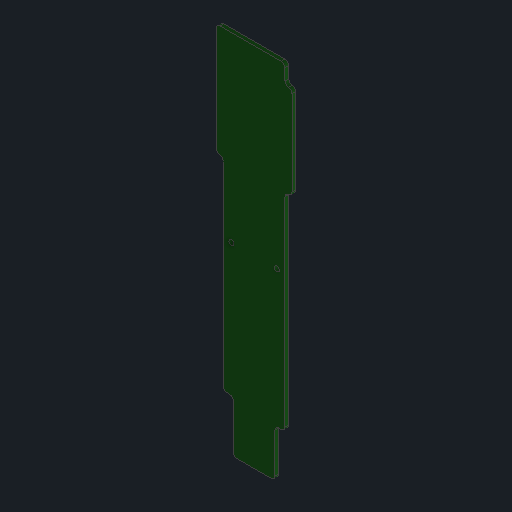
# Autodesk Inventor part: Power Board
Saved by Autodesk Inventor 2026.1 (Build 301233020, 233B)
## iProperties
Created: 2025-11-16
Part Number: Power Board
Material: Generic
Document SubType Name: Modeling
Designer: Bahaa
Density: 1 g/cm^3
Appearance: Default
Author: Bahaa
Autodesk Inventor part; units mm, degrees
ref_plane "YZ Plane" through (0, 0, 0) normal (1, 0, 0) x (0, 1, 0)
ref_plane "XZ Plane" through (0, 0, 0) normal (0, 1, 0) x (-1, 0, 0)
ref_plane "XY Plane" through (0, 0, 0) normal (0, 0, 1) x (1, 0, 0)
sketch "Sketch1" plane through (0, 0, 0) normal (0, 1, 0) x (-1, 0, 0)
  line L0 (-16.25, 55) -> (16.25, 55)
  line L1 (16.25, 55) -> (16.25, -55)
  line L2 (16.25, -55) -> (-16.25, -55)
  line L3 (-16.25, -55) -> (-16.25, 55)
  line L4 (-16.25, 55) -> (16.25, -55) construction
  line L5 (16.25, 55) -> (-16.25, -55) construction
  line L6 (16.25, 0) -> (12, 0) construction
  circle A0 centre (12, 0) radius 1.35
  line L7 (0, 0) -> (0, -55) construction
  circle A1 centre (-12, 0) radius 1.35
  line L8 (16.25, -55) -> (20, -55)
  line L9 (20, -55) -> (20, -37)
  line L10 (20, -37) -> (16.25, -37)
  line L11 (16.25, -37) -> (16.25, -55)
  line L12 (16.25, 0) -> (-16.25, 0) construction
  line L13 (0, 0) -> (0, 55) construction
  line L14 (-16.25, -55) -> (-20, -55)
  line L15 (-20, -55) -> (-20, -37)
  line L16 (-20, -37) -> (-16.25, -37)
  line L17 (-16.25, -37) -> (-16.25, -55)
  line L18 (16.25, 55) -> (-16.25, 55)
  line L19 (16.25, 55) -> (20, 55)
  line L20 (20, 55) -> (20, 37)
  line L21 (20, 37) -> (16.25, 37)
  line L22 (16.25, 37) -> (16.25, 55)
  line L23 (-20, 37) -> (-16.25, 37)
  line L24 (-16.25, 55) -> (-20, 55)
  line L25 (-20, 55) -> (-20, 37)
  line L26 (-16.25, 37) -> (-16.25, 55)
  circle A2 centre (12, 0) radius 2.55
  circle A3 centre (-12, 0) radius 2.55
  line L27 (20, 55) -> (-20, 55)
  line L28 (-20, 55) -> (-20, 90)
  line L29 (-20, 90) -> (20, 90)
  line L30 (20, 90) -> (20, 55)
  line L31 (16.25, 0) -> (-16.25, 0) construction
  line L32 (-20, -55) -> (-20, -90)
  line L33 (-20, -90) -> (20, -90)
  line L34 (20, -90) -> (20, -55)
  line L35 (16.25, -90) -> (16.25, 90)
  line L36 (-16.25, -90) -> (-16.25, 90)
  line L37 (20, -79.75) -> (-20, -79.75)
  line L38 (-11, -90) -> (11, -90)
  line L39 (11, -90) -> (11, -79.75)
  line L40 (11, -79.75) -> (-11, -79.75)
  line L41 (-11, -79.75) -> (-11, -90)
  line L42 (-11, -90) -> (11, -79.75) construction
  line L43 (11, -90) -> (-11, -79.75) construction
  line L44 (11, -87.25) -> (-11, -87.25)
  line L45 (0, 90) -> (0, 96) construction
  line L46 (20, 90) -> (-20, 90)
  line L47 (-20, 90) -> (-20, 96)
  line L48 (-20, 96) -> (20, 96)
  line L49 (20, 96) -> (20, 90)
  line L50 (-20, 90) -> (-16.25, 90)
  line L51 (-16.25, 90) -> (-16.25, 86)
  line L52 (-16.25, 86) -> (-20, 86)
  line L53 (-20, 86) -> (-20, 90)
  line L54 (-16.25, 90) -> (-16.25, 96)
  line L55 (-16.25, -79.75) -> (-11, -79.75)
  line L56 (-11, -79.75) -> (-11, -72.25)
  line L57 (-11, -72.25) -> (-16.25, -72.25)
  line L58 (-16.25, -72.25) -> (-16.25, -79.75)
  line L59 (20, 96) -> (16.25, 96)
  line L60 (16.25, 96) -> (16.25, 86)
  line L61 (16.25, 86) -> (20, 86)
  line L62 (20, 86) -> (20, 96)
  line L63 (16.25, -79.75) -> (11, -79.75)
  line L64 (11, -79.75) -> (11, -69.75)
  line L65 (11, -69.75) -> (16.25, -69.75)
  line L66 (16.25, -69.75) -> (16.25, -79.75)
  line L67 (20, -90) -> (-20, -90)
  line L68 (-20, -90) -> (-20, -97.25)
  line L69 (-20, -97.25) -> (20, -97.25)
  line L70 (20, -97.25) -> (20, -90)
  line L71 (11, -90) -> (11, -97.25)
  line L72 (-11, -90) -> (-11, -97.25)
  point P0 (16.25, 37)
  point P1 (-16.25, 37)
  point P2 (-16.25, -37)
  point P3 (16.25, -37)
  point P4 (-20, 55)
  point P5 (-20, -55)
  point P6 (0, 0)
  point P7 (0, -84.875)
  point P8 (-16.25, 86)
  point P9 (-20, 86)
  dimension "d10" = 32.5
  dimension "d11" = 110
  dimension "d16" = 2.7
  dimension "d30" = 18
  dimension "d34" = 5.1
  dimension "d35" = 40
  dimension "d36" = 35
  dimension "d39" = 40
  dimension "d40" = 24
  dimension "d41" = 10.25
  dimension "d43" = 5.125
  dimension "d45" = 2.75
  dimension "d46" = 11
  dimension "d47" = 20
  dimension "d48" = 6
  dimension "d49" = 40
  dimension "d50" = 6
  dimension "d51" = 3.75
  dimension "d52" = 4
  dimension "d53" = 5.25
  dimension "d54" = 7.5
  dimension "d55" = 3.75
  dimension "d56" = 10
  dimension "d57" = 5.25
  dimension "d58" = 10
  dimension "d59" = 7.25
  constraints: 146 end point, 20 parallel, 17 point on line, 16 symmetric about line, 15 perpendicular, 11 horizontal, 10 midpoint, 4 centre point, 2 coincident, 1 vertical, 2 other
  measures "d10" distance of L1.end L2.end
  measures "d11" distance of L0.end L1.end
  measures "d16" diameter of A0
  measures "d30" distance of L8.end L9.end
  measures "d34" diameter of A2
  measures "d35" distance of L28.end L29.end
  measures "d36" distance of L27.end L28.end
  measures "d39" diameter of L9 L7
  measures "d40" diameter of L6.end point (0, 0)
  measures "d41" distance between parallel lines of L33 L37
  measures "d43" distance from line of L33 point (0, -84.875)
  measures "d45" distance between parallel lines of L33 L44
  measures "d46" distance from line of point (0, -84.875) L39
  measures "d47" distance from line of L34 point (0, -84.875)
  measures "d48" distance of L45.start L45.end
  measures "d49" distance of L47.end L48.end
  measures "d50" distance of L48.end L29.end
  measures "d51" distance of L51.end L52.end
  measures "d52" distance of L50.end L51.end
  measures "d53" distance of L57.end L56.end
  measures "d54" distance of L56.end L55.end
  measures "d55" distance of L61.end L60.end
  measures "d56" distance of L60.end L59.end
  measures "d57" distance of L64.end L65.end
  measures "d58" distance of L63.end L64.end
  measures "d59" distance of L69.end L34.start
extrude "Extrusion1" add sketch "Sketch1" along normal blind 2 contours L36 L29 L35 L0 | L0 L1 L2 L3 | L3 L23 L25 L24 | L24 L28 L52 L36 | L19 L20 L21 L1 | L35 L61 L30 L19 | L35 L29 L30 L61 | L54 L48 L60 L29 | L60 L48 L49 L29 | L2 L35 L65 L64 L37 L56 L57 L36 | L37 L39 L44 L41 | L41 L44 L39 L33 | L33 L71 L69 L72 | A2 | A3
sketch "Sketch2" plane through (0, 0, 0) normal (0, -1, 0) x (1, 0, 0)
  line L0 (-16.25, -33.5) -> (-16.25, 37) projected
  line L1 (-16.25, -20.3135) -> (-16.25, -7.8135)
  line L2 (-16.25, -20.3135) -> (-7.5, -20.3135)
  line L3 (-7.5, -20.3135) -> (-7.5, -7.8135)
  line L4 (-7.5, -7.8135) -> (-16.25, -7.8135)
  line L5 (-16.25, -7.8135) -> (-16.25, -20.3135)
  line L6 (0, 0) -> (-16.25, 1.75) construction
  line L7 (0, 0) -> (0, 10) construction
  line L8 (0, 0) -> (-9.9425, 1.0707) construction
  line L9 (16.25, -20.3135) -> (16.25, -7.8135)
  line L10 (16.25, -20.3135) -> (7.5, -20.3135)
  line L11 (7.5, -20.3135) -> (7.5, -7.8135)
  line L12 (7.5, -7.8135) -> (16.25, -7.8135)
  line L13 (16.25, -7.8135) -> (16.25, -20.3135)
  line L14 (-11.5523, 23.3076) -> (-14.2138, 11.0942)
  line L15 (-11.5523, 23.3076) -> (-3.003, 21.4446)
  line L16 (-3.003, 21.4446) -> (-5.6644, 9.2312)
  line L17 (-5.6644, 9.2312) -> (-14.2138, 11.0942)
  line L18 (-14.2138, 11.0942) -> (-11.5523, 23.3076)
  line L19 (20.2025, 16.3879) -> (17.541, 4.1745)
  line L20 (20.2025, 16.3879) -> (11.6531, 18.2509)
  line L21 (11.6531, 18.2509) -> (8.9917, 6.0375)
  line L22 (8.9917, 6.0375) -> (17.541, 4.1745)
  line L23 (17.541, 4.1745) -> (20.2025, 16.3879)
  line L24 (-7.5, -20.3135) -> (-21.6421, -34.4557)
  line L25 (-7.5, -20.3135) -> (12.5, -20.3135) construction
  line L26 (-3.003, 21.4446) -> (-13.8098, 38.2736)
  line L27 (12.5, -20.3135) -> (21.6421, -34.4557)
  line L28 (11.6531, 18.2509) -> (13.8098, 38.2736)
  line L29 (16.25, 37) -> (16.25, -72.25) projected
  point P0 (-20, -60)
  point P1 (-20, 60)
  point P2 (-15, -60)
  point P3 (-15, 60)
  point P4 (20, 7.8135)
  point P5 (20, -7.8135)
  point P6 (-16.25, 20.3135)
  point P7 (-16.25, 7.8135)
  point P8 (-16.25, -7.8135)
  point P9 (15, 7.8135)
  point P10 (15, -7.8135)
  point P11 (-16.25, 37)
  point P12 (16.25, -33.5)
  point P13 (16.25, 7.8135)
  point P14 (16.25, -90)
  point P15 (16.25, -79.75)
  point P16 (17.9687, 1.4962)
  point P17 (-12.3889, 13.1007)
  dimension "d18" = 12.5
  dimension "d19" = 7.8135
  dimension "d20" = 10
  dimension "d21" = 10
  dimension "d25" = 15
  dimension "d37" = 20
  dimension "d38" = 135
  constraints: 56 end point, 18 symmetric about line, 2 horizontal, 2 parallel, 1 equal length, 1 perpendicular, 1 point on line, 1 vertical, 5 other
  measures "d18" distance between parallel lines of L2 L4
  measures "d19" distance from line of L6.start L4
  measures "d20" distance of L6.start L7.end
  measures "d21" distance of L6.start L8.end
  measures "d25" distance between parallel lines of L11 L3
  measures "d37" distance of L2.end L24.end
  measures "d38" angle of L24 L25
extrude "Extrusion2" [suppressed]
fillet "Fillet2" radius 2 14 edges at (16.25, 1, 37) (20, 1, 37) (-20, 1, 37) (-16.25, 1, 37) (-20, 1, 96) (16.25, 1, 96) (16.25, 1, 86) (20, 1, 86) (11, 1, -72.25) (16.25, 1, -72.25) (-16.25, 1, -69.75) (-11, 1, -69.75) (11, 1, -97.25) (-11, 1, -97.25)
chamfer "Chamfer1" [suppressed]
fillet "Fillet3" [suppressed]
fillet "Fillet5" [suppressed]
body "Solid1"
